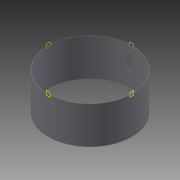
# Autodesk Inventor part: Cyclone Main Straight Metal
Saved by Autodesk Inventor 2018.2 (Build 222227000, 227)
## iProperties
Created: 2018-02-08
Part Number: Cyclone Main Straight Metal
Material: Generic
Document SubType Name: Modeling
Designer: Rus
Density: 1 g/cm^3
Appearance: Default
Author: Rus
Autodesk Inventor part; units mm, degrees
ref_plane "YZ Plane" through (0, 0, 0) normal (1, 0, 0) x (0, 1, 0)
ref_plane "XZ Plane" through (0, 0, 0) normal (0, 1, 0) x (-1, 0, 0)
ref_plane "XY Plane" through (0, 0, 0) normal (0, 0, 1) x (1, 0, 0)
sketch "Sketch1" plane through (0, 0, 0) normal (0, 1, 0) x (-1, 0, 0)
  circle A0 centre (0, 0) radius 228.6
  circle A1 centre (0, 0) radius 227.5764
  line L0 (0, 0) -> (0, 228.6) construction
  line L1 (0, 0) -> (-228.6, 0) construction
  line L2 (0, 0) -> (228.6, 0) construction
  line L3 (0, 0) -> (0, -228.6) construction
  dimension "d0" = 1.0236
  dimension "d1" = 457.2
  constraints: 8 end point, 4 point on circle, 2 centre point, 2 coincident, 2 horizontal, 2 vertical
  measures "d0" radial gap between concentric circles of A0 A1
  measures "d1" diameter of A0
ref_plane "Work Plane1" through (0, 0, 228.6) normal (0, 0, 1) x (1, 0, 0)
ref_plane "Work Plane2" through (-228.6, 0, 0) normal (-1, 0, 0) x (0, -1, 0)
ref_plane "Work Plane3" through (0, 0, -228.6) normal (0, 0, -1) x (-1, 0, 0)
ref_plane "Work Plane4" through (228.6, 0, 0) normal (1, 0, 0) x (0, 1, 0)
extrude "Extrusion1" add sketch "Sketch1" against normal blind 203.2
sketch "Sketch2" plane through (0, 0, -228.6) normal (0, 0, -1) x (-1, 0, 0)
  line L0 (-228.6, -203.2) -> (228.6, -203.2) construction
  line L1 (0, 0) -> (0, -50.8) construction
  line L2 (0, -127) -> (0, -50.8) construction
  line L3 (0, -127) -> (25.4, -127)
  line L4 (25.4, -127) -> (25.4, -50.8)
  line L5 (25.4, -50.8) -> (0, -50.8)
  line L6 (0, -127) -> (0, -50.8)
  line L7 (-228.6, 0) -> (-228.6, -203.2) projected
  point P0 (228.6, 0)
  dimension "d4" = 50.8
  dimension "d9" = 76.2
  dimension "d10" = 25.4
  constraints: 12 end point, 2 horizontal, 1 parallel, 1 vertical
  measures "d4" distance of L1.start L1.end
  measures "d9" distance of L3.end L4.end
  measures "d10" distance between parallel lines of L4 L2
extrude "Extrusion2" cut sketch "Sketch2" against normal blind 228.6
body "Solid1"
